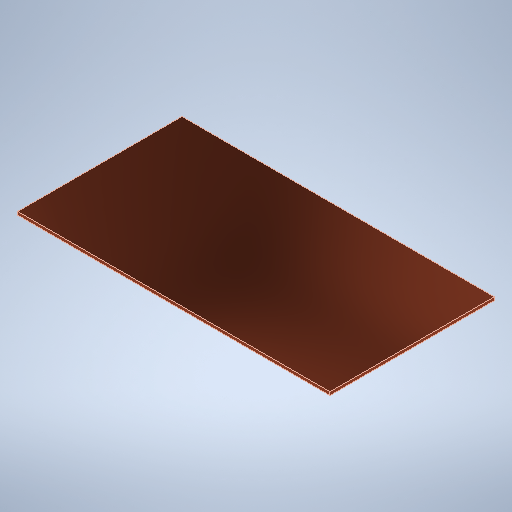
# Autodesk Inventor part: bakelite
Saved by Autodesk Inventor 2025 (Build 290162000, 162)
## iProperties
Created: 2024-09-26
Part Number: bakelite
Material: Copper
Document SubType Name: Modeling
Designer: DANIEL
Density: 8.94 g/cm^3
Appearance: Copper - Polished
Author: DANIEL
Autodesk Inventor part; units mm, degrees
ref_plane "YZ Plane" through (0, 0, 0) normal (1, 0, 0) x (0, 1, 0)
ref_plane "XZ Plane" through (0, 0, 0) normal (0, 1, 0) x (-1, 0, 0)
ref_plane "XY Plane" through (0, 0, 0) normal (0, 0, 1) x (1, 0, 0)
sketch "Sketch1" plane through (0, 0, 0) normal (0, 1, 0) x (-1, 0, 0)
  line L0 (47.5, 25) -> (-47.5, 25)
  line L1 (-47.5, 25) -> (-47.5, -25)
  line L2 (-47.5, -25) -> (47.5, -25)
  line L3 (47.5, -25) -> (47.5, 25)
  line L4 (47.5, 25) -> (-47.5, -25) construction
  line L5 (-47.5, 25) -> (47.5, -25) construction
  point P0 (0, 0)
  dimension "d0" = 95
  dimension "d1" = 50
  constraints: 12 end point, 2 midpoint, 2 parallel, 1 horizontal, 1 perpendicular
  measures "d0" distance of L2.end L1.end
  measures "d1" distance of L1.end L0.end
extrude "Extrusion1" add sketch "Sketch1" along normal blind 1
body "Solid1"
